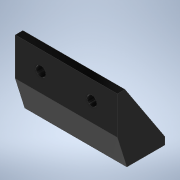
# Autodesk Inventor part: Soporte Cajas
Saved by Autodesk Inventor 2020.3 (Build 243373000, 373)
## iProperties
Created: 2021-04-28
Part Number: Soporte Cajas
Material: PET Plastic
Document SubType Name: Modeling
Designer: juanp
Density: 1.541 g/cm^3
Appearance: Polycarbonate - Clear
Author: juanp
Autodesk Inventor part; units mm, degrees
ref_plane "YZ Plane" through (0, 0, 0) normal (1, 0, 0) x (0, 1, 0)
ref_plane "XZ Plane" through (0, 0, 0) normal (0, 1, 0) x (-1, 0, 0)
ref_plane "XY Plane" through (0, 0, 0) normal (0, 0, 1) x (1, 0, 0)
sketch "Sketch7" plane through (0, 0, 0) normal (1, 0, 0) x (0, 1, 0)
  line L0 (36, 0) -> (36, -4)
  line L1 (36, -4) -> (4, -25)
  line L2 (4, -25) -> (0, -25)
  line L3 (0, -25) -> (0, 0)
  line L4 (0, 0) -> (36, 0)
  line L5 (36, -4) -> (16.6104, -4)
  line L6 (4, -7.9408) -> (4, -25)
  line L7 (16, 0) -> (0, -5)
  line L8 (4, -7.9408) -> (16.6104, -4)
  dimension "d35" = 4
  dimension "d36" = 25
  dimension "d37" = 36
  dimension "d43" = 4
  dimension "d44" = 20
  dimension "d45" = 20
  constraints: 18 end point, 4 perpendicular, 2 point on line, 2 vertical, 1 horizontal, 1 parallel
  measures "d35" distance of L0.start L0.end
  measures "d36" distance of L2.end L3.end
  measures "d37" distance of L3.end L0.start
  measures "d43" distance between parallel lines of L8 L7
  measures "d44" distance of L0.start L7.start
  measures "d45" distance of L2.end L7.end
extrude "Extrusion6" add sketch "Sketch7" along normal mid plane 54 contours L0 L5 L8 L6 L2 L3 L7 L4
sketch "Sketch8" plane through (27, 36, -4) normal (0, 0, -1) x (-1, 0, 0)
  line L0 (0, -10) -> (13.5, -10) construction
  line L1 (13.5, -10) -> (27, -10) construction
  line L2 (27, -10) -> (40.5, -10) construction
  line L3 (40.5, -10) -> (54, -10) construction
  circle A0 centre (13.5, -10) radius 2.65
  circle A1 centre (40.5, -10) radius 2.65
  line L4 (0, -19.3896) -> (0, 0) projected
  line L5 (54, 0) -> (54, -19.3896) projected
  line L6 (54, 0) -> (0, 0) projected
  point P0 (27, -36)
  dimension "d46" = 5.3
  dimension "d55" = 10
  constraints: 8 end point, 5 point on line, 3 collinear, 2 centre point, 2 coincident, 1 equal radius, 1 horizontal
  measures "d46" diameter of A1
  measures "d55" distance between parallel lines of L6 L1
extrude "Extrusion7" cut sketch "Sketch8" against normal through all
sketch "Sketch9" plane through (-27, 4, -7.9408) normal (0, 1, 0) x (1, 0, 0)
  line L0 (54, 17.0592) -> (54, 0) projected
  line L1 (54, 8.5296) -> (40.5, 8.5296) construction
  line L2 (40.5, 8.5296) -> (27, 8.5296) construction
  line L3 (27, 8.5296) -> (13.5, 8.5296) construction
  line L4 (13.5, 8.5296) -> (0, 8.5296) construction
  line L5 (0, 0) -> (0, 17.0592) projected
  circle A0 centre (40.5, 8.5296) radius 2.65
  circle A1 centre (13.5, 8.5296) radius 2.65
  point P0 (27, -7.9408)
  dimension "d49" = 5.3
  constraints: 8 end point, 3 collinear, 2 centre point, 2 coincident, 2 midpoint, 2 point on line, 1 equal radius, 1 horizontal
  measures "d49" diameter of A1
extrude "Extrusion8" cut sketch "Sketch9" against normal blind 10
ref_plane "Work Plane4" through (0, 4, -25) normal (0, 0.5486564, -0.8360479) x (-1, 0, 0)
sketch "Sketch10" plane through (0, 4, -25) normal (0, 0.5486564, -0.8360479) x (-1, 0, 0)
  line L0 (-27, 38.2753) -> (-25, 38.2753)
  line L1 (-25, 38.2753) -> (-25, 0)
  line L2 (-25, 0) -> (-27, 0)
  line L3 (-27, 0) -> (-27, 38.2753)
  line L4 (27, 0) -> (25, 0)
  line L5 (25, 0) -> (25, 38.2753)
  line L6 (25, 38.2753) -> (27, 38.2753)
  line L7 (27, 38.2753) -> (27, 0)
  line L8 (-1, 38.2753) -> (1, 38.2753)
  line L9 (1, 38.2753) -> (1, 0)
  line L10 (1, 0) -> (-1, 0)
  line L11 (-1, 0) -> (-1, 38.2753)
  line L12 (27, 38.2753) -> (-27, 38.2753) projected
  line L13 (-27, 0) -> (27, 0) projected
  point P0 (0, 10.3722)
  point P1 (0, 38.2753)
  dimension "d52" = 2
  constraints: 24 end point, 8 parallel, 3 collinear, 3 horizontal, 3 perpendicular, 3 point on line, 2 midpoint
  measures "d52" distance between parallel lines of L7 L5
extrude "Extrusion9" add sketch "Sketch10" against normal up to next contours L0 L1 L2 L3 | L8 L9 L10 L11 | L6 L7 L4 L5
body "Solid2"
